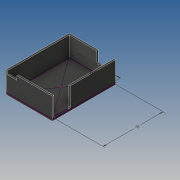
# Autodesk Inventor part: housing-lvl-bottom
Saved by Autodesk Inventor 2018.3 (Build 223284000, 284)
## iProperties
Manager: feesmrt
Company: FRANCOR
Part Number: housing-lvl-bottom
Project: Rescue Robot
Cost Center: -
Material: ABS-Kunststoff
Document SubType Name: Modeling
Designer: feesmrt
Engineer: feesmrt
Authority: feesmrt
Density: 1.06 g/cm^3
Appearance: Glatt - schwarz
Subject: Rescue Robot
Author: feesmrt
Revision Number: 1
Autodesk Inventor part; units mm, degrees
ref_plane "YZ Plane" through (0, 0, 0) normal (1, 0, 0) x (0, 1, 0)
ref_plane "XZ Plane" through (0, 0, 0) normal (0, 1, 0) x (-1, 0, 0)
ref_plane "XY Plane" through (0, 0, 0) normal (0, 0, 1) x (1, 0, 0)
sketch "Skizze1" plane through (0, 0, 0) normal (0, 0, 1) x (1, 0, 0)
  line L0 (-27.25, -38) -> (27.25, -38)
  line L1 (27.25, -38) -> (27.25, 38)
  line L2 (27.25, 38) -> (-27.25, 38)
  line L3 (-27.25, 38) -> (-27.25, -38)
  line L4 (-27.25, -38) -> (27.25, 38) construction
  line L5 (27.25, -38) -> (-27.25, 38) construction
  line L6 (-29.25, -40) -> (29.25, -40)
  line L7 (29.25, -40) -> (29.25, 40)
  line L8 (29.25, 40) -> (-29.25, 40)
  line L9 (-29.25, 40) -> (-29.25, -40)
  line L10 (-29.25, -40) -> (29.25, 40) construction
  line L11 (29.25, -40) -> (-29.25, 40) construction
  point P0 (0, 0)
  dimension "d0" = 54.5
  dimension "d1" = 76
  dimension "d2" = 2
  dimension "d3" = 2
  constraints: 24 end point, 4 midpoint, 4 parallel, 2 horizontal, 2 perpendicular
  measures "d0" distance of L1.end L2.end
  measures "d1" distance of L0.end L1.end
  measures "d2" distance between parallel lines of L7 L1
  measures "d3" distance between parallel lines of L8 L2
extrude "Extrusion1" add sketch "Skizze1" against normal blind 2.5 contours L3 L2 L1 L0 | L9 L8 L7 L6
extrude "Extrusion2" add sketch "Skizze1" along normal blind 25
sketch "Skizze2" plane through (0, 0, 25) normal (0, 0, 1) x (1, 0, 0)
  line L0 (27.25, -38) -> (-27.25, -38) projected
  line L1 (27.25, 38) -> (27.25, -38) projected
  line L2 (29.25, -40) -> (29.25, 40) projected
  line L3 (29.25, 40) -> (-29.25, 40) projected
  line L4 (-27.25, 38) -> (27.25, 38) projected
  line L5 (-29.25, -40) -> (29.25, -40) projected
  line L6 (27.25, -38) -> (27.25, 38) projected
  line L7 (29.25, 40) -> (29.25, -40) projected
  line L8 (27.25, -38) -> (29.25, -38)
  line L9 (29.25, -38) -> (29.25, -17)
  line L10 (29.25, -17) -> (27.25, -17)
  line L11 (27.25, -17) -> (27.25, -38)
  point P0 (0, 0)
  dimension "d8" = 21
  constraints: 8 end point, 2 parallel, 1 horizontal, 1 perpendicular, 1 point on line
  measures "d8" distance between parallel lines of L8 L10
extrude "Extrusion3" cut sketch "Skizze2" against normal up to surface (25 mm away)
sketch "Skizze3" plane through (0, 0, 25) normal (0, 0, 1) x (1, 0, 0)
  line L0 (-27.25, 38) -> (27.25, 38) projected
  line L1 (29.25, 40) -> (-29.25, 40) projected
  line L2 (27.25, 38) -> (27.25, -17) projected
  line L3 (27.25, 38) -> (7.25, 38)
  line L4 (7.25, 38) -> (7.25, 40)
  line L5 (7.25, 40) -> (27.25, 40)
  line L6 (27.25, 40) -> (27.25, 38)
  point P0 (0, 0)
  dimension "d11" = 20
  constraints: 8 end point, 2 parallel, 1 horizontal, 1 perpendicular, 1 point on line
  measures "d11" distance between parallel lines of L6 L4
extrude "Extrusion4" cut sketch "Skizze3" against normal blind 15
chamfer "Fase1" distance 1.5 angle 45 4 edges at (28.25, -17, 0) (1, -38, 0) (7.25, 39, 10) (27.25, 39, 10)
sketch "Skizze4" plane through (0, 0, 25) normal (0, 0, 1) x (1, 0, 0)
  line L0 (-27.25, -38) -> (-27.25, 38) projected
  line L1 (29.25, -38) -> (-27.25, -38) projected
  line L2 (-29.25, -40) -> (29.25, -40) projected
  line L3 (-27.25, -38) -> (29.25, -38) projected
  line L4 (-27.25, -38) -> (-27.25, -40)
  line L5 (29.25, -40) -> (-29.25, -40) projected
  line L6 (-27.25, -40) -> (-15.5394, -40)
  line L7 (-15.5394, -38) -> (-15.5394, -40)
  line L8 (-15.5394, -38) -> (-27.25, -38)
  point P0 (0, 0)
  dimension "d17" = 11.7106
  constraints: 8 end point, 3 point on line, 2 perpendicular, 1 vertical
  measures "d17" distance between parallel lines of L4 L7
extrude "Extrusion5" cut sketch "Skizze4" against normal blind 5
equation "\"d3\" = d2"
